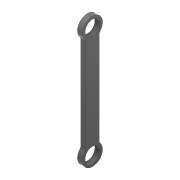
# Autodesk Inventor part: Cursor
Saved by Autodesk Inventor 2020 (Build 240168000, 168)
## iProperties
Created: 2021-09-22
Part Number: Cursor
Material: Generic
Document SubType Name: Modeling
Designer: pablo
Density: 1 g/cm^3
Appearance: Smooth - Black
Author: pablo
Autodesk Inventor part; units mm, degrees
ref_plane "YZ Plane" through (0, 0, 0) normal (1, 0, 0) x (0, 1, 0)
ref_plane "XZ Plane" through (0, 0, 0) normal (0, 1, 0) x (-1, 0, 0)
ref_plane "XY Plane" through (0, 0, 0) normal (0, 0, 1) x (1, 0, 0)
sketch "Sketch1" plane through (0, 0, 0) normal (1, 0, 0) x (0, 1, 0)
  circle A0 centre (0, 0) radius 10
  circle A1 centre (0, 0) radius 7.5
  line L0 (0, -6.5) -> (110, -6.5)
  line L1 (9.0104, 0) -> (0, 0)
  line L2 (0, 6.5) -> (110, 6.5)
  circle A2 centre (110, 0) radius 10
  circle A3 centre (110, 0) radius 7.5
  line L3 (119.0104, 0) -> (110, 0)
  point P0 (110, 6.5)
  point P1 (7.5993, -6.5)
  point P2 (102.4007, -6.5)
  point P3 (102.4007, 6.5)
  point P4 (7.5993, 6.5)
  dimension "d0" = 20
  dimension "d1" = 15
  dimension "d4" = 110
  dimension "d5" = 6.5
  dimension "d8" = 110
  constraints: 8 end point, 4 centre point, 4 coincident, 3 horizontal, 2 symmetric about line, 9 other
  measures "d0" diameter of A0
  measures "d1" diameter of A1
  measures "d4" distance of L0.start L0.end
  measures "d5" distance of point (0, 0) L0.start
  measures "d8" distance of point (0, 0) point (110, 0)
extrude "Extrusion1" add sketch "Sketch1" along normal blind 5 contours A0 L0 A1 L2 | A0 L2 A2 L0 | L2 A1 L0 A0 | A2 L0 A3 L2 | L2 A3 L0 A2
fillet "Fillet1" radius 4 4 edges at (2.5, 102.4007, 6.5) (2.5, 102.4007, -6.5) (2.5, 7.5993, -6.5) (2.5, 7.5993, 6.5)
body "Solid1"
